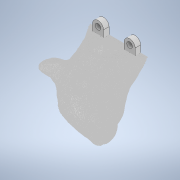
# Autodesk Inventor part: squirrel_head_lg
Saved by Autodesk Inventor 2020 (Build 240168000, 168)
## iProperties
Created: 2019-05-04
Part Number: squirrel_head_lg
Material: Generic
Document SubType Name: Modeling
Designer: mfans
Density: 1 g/cm^3
Appearance: Default
Author: mfans
Autodesk Inventor part; units mm, degrees
ref_plane "YZ Plane" through (0, 0, 0) normal (1, 0, 0) x (0, 1, 0)
ref_plane "XZ Plane" through (0, 0, 0) normal (0, 1, 0) x (-1, 0, 0)
ref_plane "XY Plane" through (0, 0, 0) normal (0, 0, 1) x (1, 0, 0)
sketch "Sketch1" plane through (20.1821, 23.0698, 0) normal (0, 0, -1) x (-1, 0, 0)
  line L0 (39.44, 3.9041) -> (-2.3601, 3.9041) projected
  line L1 (3.6821, 3.9041) -> (9.6821, 3.9041)
  line L2 (9.6821, 3.9041) -> (9.6821, 11.9041)
  line L3 (9.6821, 11.9041) -> (3.6821, 11.9041)
  line L4 (3.6821, 11.9041) -> (3.6821, 3.9041)
  line L5 (26.6821, 3.9041) -> (32.6821, 3.9041)
  line L6 (32.6821, 3.9041) -> (32.6821, 11.9041)
  line L7 (32.6821, 11.9041) -> (26.6821, 11.9041)
  line L8 (26.6821, 11.9041) -> (26.6821, 3.9041)
  point P0 (20.1821, -23.0698)
  point P1 (9.6821, 3.9041)
  dimension "d0" = 6
  dimension "d1" = 8
  dimension "d2" = 17
  dimension "d3" = 6.5
  constraints: 16 end point, 4 parallel, 3 point on line, 2 horizontal, 2 perpendicular, 1 collinear
  measures "d0" distance of L6.end L7.end
  measures "d1" distance of L5.end L6.end
  measures "d2" distance between parallel lines of L2 L8
  measures "d3" distance from line of point (20.182, -23.07) L8
extrude "Extrusion1" add sketch "Sketch1" against normal blind 4
fillet "Fillet1" radius 3 4 edges at (16.5, 34.9739, 2) (10.5, 34.9739, 2) (-6.5, 34.9739, 2) (-12.5, 34.9739, 2)
thicken "Thicken1" operation add thickness 1 both sides no extend neighbours yes toward (0, 1, 0) faces at (13.5, 34.9739, 1.3333) (10.9019, 33.474, 1.3333) (16.0981, 33.474, 1.3333)
thicken "Thicken2" operation add thickness 1 both sides no extend neighbours yes toward (0, 1, 0) faces at (-9.5, 34.9739, 1.3333) (-12.0981, 33.474, 1.3333) (-6.9019, 33.474, 1.3333)
sketch "Sketch2" plane through (20.1821, 23.0698, 4) normal (0, 0, 1) x (1, 0, 0)
  arc A0 (-2.6821, 8.9041) -> (-10.6821, 8.9041) centre (-6.6821, 8.9041) ccw projected
  line L0 (-10.6821, 8.9041) -> (-10.6821, 3.9041) projected
  line L1 (-10.6821, 3.9041) -> (-2.6821, 3.9041) projected
  line L2 (-2.6821, 3.9041) -> (-2.6821, 8.9041) projected
  arc A1 (-25.6821, 8.9041) -> (-33.6821, 8.9041) centre (-29.6821, 8.9041) ccw projected
  line L3 (-33.6821, 8.9041) -> (-33.6821, 3.9041) projected
  line L4 (-33.6821, 3.9041) -> (-25.6821, 3.9041) projected
  line L5 (-25.6821, 3.9041) -> (-25.6821, 8.9041) projected
  point P0 (-20.1821, -23.0698)
  constraints: 2 coincident
hole "Hole1" at (13.5, 31.9739, 4) at (-9.5, 31.9739, 4) direction (0, 0, -1) diameter 4 end through all
body "Solid1"
